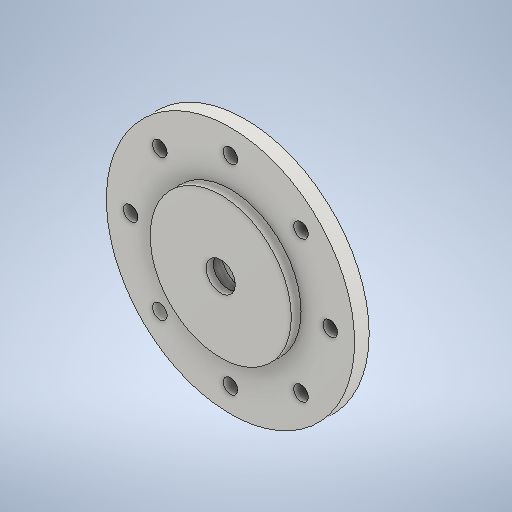
# Autodesk Inventor part: 08 CYLINDER REAR COVER
Saved by Autodesk Inventor 2025.2 (Build 292293000, 293)
## iProperties
Created: 2025-05-29
Part Number: 08 CYLINDER REAR COVER
Material: Steel AISI 1020 107 HR
Document SubType Name: Modeling
Designer: bless
Density: 7.87 g/cm^3
Appearance: Steel
Author: bless
Autodesk Inventor part; units mm, degrees
ref_plane "YZ Plane" through (0, 0, 0) normal (1, 0, 0) x (0, 1, 0)
ref_plane "XZ Plane" through (0, 0, 0) normal (0, 1, 0) x (-1, 0, 0)
ref_plane "XY Plane" through (0, 0, 0) normal (0, 0, 1) x (1, 0, 0)
sketch "Sketch1" plane through (0, 0, 0) normal (0, 0, 1) x (1, 0, 0)
  circle A0 centre (0, 0) radius 25.5
  dimension "d0" = 51
  constraints: 1 centre point, 1 coincident
  measures "d0" diameter of A0
extrude "Extrusion1" add sketch "Sketch1" along normal blind 3
sketch "Sketch2" plane through (0, 0, 3) normal (0, 0, 1) x (1, 0, 0)
  circle A0 centre (0, 0) radius 25.5 projected
  circle A1 centre (0, 0) radius 14.5
  dimension "d3" = 29
  constraints: 1 centre point, 1 coincident
  measures "d3" diameter of A1
extrude "Extrusion2" add sketch "Sketch2" along normal blind 2 contours A1
sketch "Sketch3" plane through (0, 0, 0) normal (0, 0, -1) x (-1, 0, 0)
  circle A0 centre (0, 0) radius 25.5 projected
  circle A1 centre (0, 0) radius 8
  dimension "d6" = 16
  constraints: 1 centre point, 1 coincident
  measures "d6" diameter of A1
extrude "Extrusion3" add sketch "Sketch3" along normal blind 9.5 contours A1
sketch "Sketch4" plane through (0, 0, 5) normal (0, 0, 1) x (1, 0, 0)
  circle A0 centre (0, 0) radius 14.5 projected
  circle A1 centre (0, 0) radius 3
  dimension "d9" = 6
  constraints: 1 centre point, 1 coincident
  measures "d9" diameter of A1
extrude "Extrusion4" cut sketch "Sketch4" against normal through all contours A1
sketch "Sketch5" plane through (0, 0, 3) normal (0, 0, 1) x (1, 0, 0)
  circle A0 centre (0, 0) radius 25.5 projected
  circle A1 centre (0, 0) radius 20.5
  circle A2 centre (0, 20.5) radius 1.5
  circle A3 centre (-14.4957, 14.4957) radius 1.5
  circle A4 centre (-20.5, 0) radius 1.5
  circle A5 centre (-14.4957, -14.4957) radius 1.5
  circle A6 centre (0, -20.5) radius 1.5
  circle A7 centre (14.4957, -14.4957) radius 1.5
  circle A8 centre (20.5, 0) radius 1.5
  circle A9 centre (14.4957, 14.4957) radius 1.5
  dimension "d12" = 41
  dimension "d13" = 3
  dimension "d16" = 360
  constraints: 8 centre point, 2 vertical alignment, 1 coincident, 19 other
  measures "d13" diameter of A2
extrude "Extrusion5" cut sketch "Sketch5" against normal through all contours A1 A8 | A1 A8 | A9 A1 | A1 A9 | A7 A1 | A1 A7 | A2 A1 | A1 A2 | A6 A1 | A1 A6 | A3 A1 | A1 A3 | A5 A1 | A1 A5 | A4 A1 | A1 A4
sketch "Sketch6" plane through (0, 0, -9.5) normal (0, 0, -1) x (-1, 0, 0)
  circle A0 centre (0, 0) radius 3 projected
hole "Hole1" at (0, 0, -9.5) direction (0, 0, 1) diameter 8.9175 depth 13 counterbore diameter 9 counterbore depth 10 thread size "M10x1" class "6H" standard "ANSI Metric M Profile"
body "Solid1"
